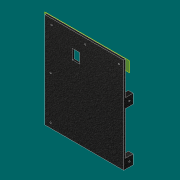
# Autodesk Inventor part: Lateral Derecho
Saved by Autodesk Inventor 2019 (Build 230136000, 136)
## iProperties
Created: 2024-12-30
Part Number: Lateral Derecho
Material: Nylon 6/6
Document SubType Name: Modeling
Designer: Familia CS
Density: 1.13 g/cm^3
Appearance: Black Cast
Author: Familia CS
Autodesk Inventor part; units mm, degrees
ref_plane "YZ Plane" through (0, 0, 0) normal (1, 0, 0) x (0, 1, 0)
ref_plane "XZ Plane" through (0, 0, 0) normal (0, 1, 0) x (-1, 0, 0)
ref_plane "XY Plane" through (0, 0, 0) normal (0, 0, 1) x (1, 0, 0)
ref_plane "Work Plane1" through (0, 0, 0) normal (0, 0, 1) x (1, 0, 0)
sketch "Sketch1" plane through (0, 0, 0) normal (0, 0, 1) x (1, 0, 0)
  line L0 (-2, -98) -> (8, -98) projected
  line L1 (-2, -98) -> (-2, 2) projected
  circle A0 centre (4, -93) radius 0.75 projected
  circle A1 centre (4, -48) radius 0.75 projected
  circle A2 centre (5, -4) radius 0.75 projected
  line L2 (0, 2) -> (80.5, 2) projected
  circle A3 centre (40.25, -4) radius 0.75 projected
  circle A4 centre (75.5, -4) radius 0.75 projected
  line L3 (34.223, -24.7194) -> (34.223, -14.2194)
  line L4 (26.723, -24.7194) -> (34.223, -24.7194)
  line L5 (26.723, -14.2194) -> (26.723, -24.7194)
  line L6 (34.223, -14.2194) -> (26.723, -14.2194)
  line L7 (80.5, 2) -> (-2, 2)
  line L8 (-2, 2) -> (-2, -98)
  line L9 (-2, -98) -> (80.5, -98)
  line L10 (80.5, -98) -> (80.5, 2)
  point P0 (0, 0)
  point P1 (20.6901, -14.1894)
  constraints: 16 end point, 3 horizontal, 2 parallel, 2 vertical, 1 perpendicular, 5 other
extrude "Extrusion1" add sketch "Sketch1" along normal blind 2
sketch "Sketch2" plane through (0, 0, 0) normal (0, 0, -1) x (-1, 0, 0)
  point P0 (0, 0)
sketch "Sketch3" plane through (0, 0, 0) normal (0, 0, -1) x (-1, 0, 0)
  point P0 (0, 0)
sketch "Sketch4" plane through (80.5, -98, 0) normal (1, 0, 0) x (0, 0, -1)
  line L0 (0, 45) -> (0, 55) projected
  line L1 (0, 45) -> (5, 45) projected
  line L2 (5, 55) -> (5, 45) projected
  line L3 (0, 55) -> (5, 55) projected
  line L4 (0, 45) -> (8, 45)
  line L5 (8, 45) -> (8, 55)
  line L6 (8, 55) -> (0, 55)
  circle A0 centre (4, 50) radius 0.75
  point P0 (0, 98)
  dimension "d3" = 8
  dimension "d4" = 10
  dimension "d6" = 1.5
  constraints: 6 end point, 1 centre point, 1 horizontal, 1 perpendicular
  measures "d3" distance of L0.start L4.end
  measures "d4" distance of L4.end L5.end
  measures "d6" diameter of A0
extrude "Extrusion2" add sketch "Sketch4" against normal blind 5
sketch "Sketch5" plane through (80.5, -98, 2) normal (1, 0, 0) x (0, 0, -1)
  line L0 (2, 45) -> (2, 0) projected
  line L1 (2, 0) -> (10, 0)
  line L2 (10, 0) -> (10, 10)
  line L3 (10, 10) -> (2, 10)
  line L4 (2, 10) -> (2, 0)
  circle A0 centre (6, 5) radius 0.75
  point P0 (2, 98)
  dimension "d9" = 8
  dimension "d10" = 10
  dimension "d12" = 1.5
  constraints: 8 end point, 2 parallel, 1 centre point, 1 horizontal, 1 perpendicular
  measures "d9" distance of L3.end L2.end
  measures "d10" distance of L2.end L1.end
  measures "d12" diameter of A0
extrude "Extrusion3" add sketch "Sketch5" against normal blind 5
sketch "Sketch6" plane through (-2, -98, 2) normal (0, -1, 0) x (1, 0, 0)
  line L0 (77.5, -10) -> (77.5, -2) projected
  line L1 (77.5, -10) -> (67.5, -10)
  line L2 (67.5, -10) -> (67.5, -2)
  line L3 (67.5, -2) -> (77.5, -2)
  line L4 (77.5, -2) -> (77.5, -10)
  circle A0 centre (72.5, -6) radius 0.75
  point P0 (2, -2)
  dimension "d15" = 10
  dimension "d16" = 8
  dimension "d18" = 1.5
  constraints: 8 end point, 2 parallel, 1 centre point, 1 horizontal, 1 perpendicular
  measures "d15" distance of L2.end L3.end
  measures "d16" distance of L1.end L2.end
  measures "d18" diameter of A0
extrude "Extrusion4" add sketch "Sketch6" against normal blind 5
sketch "Sketch7" plane through (-2, -98, 2) normal (0, -1, 0) x (1, 0, 0)
  line L0 (10, -2) -> (10, -17) projected
  line L1 (67.5, -10) -> (67.5, -2) projected
  circle A0 centre (32.473, -6) radius 0.75
  line L2 (32.473, -10) -> (27.473, -10)
  line L3 (27.473, -10) -> (27.473, -2)
  line L4 (27.473, -2) -> (37.473, -2)
  line L5 (37.473, -2) -> (37.473, -10)
  line L6 (37.473, -10) -> (32.473, -10)
  point P0 (2, -2)
  dimension "d22" = 1.5
  dimension "d25" = 4
  dimension "d26" = 5
  dimension "d27" = 8
  dimension "d28" = 10
  dimension "d29" = 8
  constraints: 10 end point, 2 perpendicular, 1 centre point, 1 point on line
  measures "d22" diameter of A0
  measures "d25" distance of A0.centre L2.start
  measures "d26" distance of L2.start L2.end
  measures "d27" distance of L2.end L3.end
  measures "d28" distance of L3.end L4.end
  measures "d29" distance of L4.end L5.end
extrude "Extrusion5" add sketch "Sketch7" against normal blind 5
sketch "Sketch8" plane through (-2, -98, 2) normal (0, -1, 0) x (1, 0, 0)
  line L0 (37.473, -10) -> (27.473, -10) projected
  line L1 (27.473, -10) -> (37.473, -10)
  line L2 (37.473, -10) -> (37.473, -2)
  line L3 (37.473, -2) -> (27.473, -2)
  line L4 (27.473, -2) -> (27.473, -10)
  point P0 (2, -2)
  constraints: 8 end point, 2 parallel, 1 horizontal, 1 perpendicular
extrude "Extrusion6" cut sketch "Sketch8" against normal blind 5
sketch "Sketch9" plane through (-2, -98, 2) normal (0, -1, 0) x (1, 0, 0)
  line L0 (47.25, -2) -> (47.25, -7) projected
  line L1 (47.25, -7) -> (37.25, -7) projected
  line L2 (37.25, -7) -> (37.25, -2) projected
  line L3 (37.25, -2) -> (47.25, -2)
  line L4 (67.5, -2) -> (0, -2) projected
  line L5 (37.25, -2) -> (37.25, -10)
  line L6 (37.25, -10) -> (47.25, -10)
  line L7 (47.25, -10) -> (47.25, -2)
  line L8 (47.25, -2) -> (37.25, -2)
  circle A0 centre (42.25, -6) radius 0.75
  point P0 (2, -2)
  dimension "d35" = 8
  dimension "d36" = 10
  dimension "d38" = 1.5
  constraints: 10 end point, 2 collinear, 1 centre point, 1 perpendicular, 1 vertical
  measures "d35" distance of L2.end L5.end
  measures "d36" distance of L5.end L6.end
  measures "d38" diameter of A0
extrude "Extrusion7" add sketch "Sketch9" against normal blind 5
sketch "Sketch10" plane through (80.5, -53, -8) normal (0, 0, -1) x (-1, 0, 0)
  line L0 (5, 10) -> (5, 0) projected
  line L1 (0, -45) -> (0, 55) projected
  line L2 (5, 0) -> (0, 0)
  line L3 (0, 0) -> (0, 10)
  line L4 (0, 10) -> (5, 10)
  line L5 (5, 10) -> (5, 0)
  point P0 (80.5, 53)
  dimension "d41" = 10
  constraints: 8 end point, 2 parallel, 1 horizontal, 1 perpendicular, 1 point on line
  measures "d41" distance of L2.end L3.end
extrude "Extrusion8" cut sketch "Sketch10" against normal blind 8
sketch "Sketch11" plane through (0, 0, 0) normal (0, 0, -1) x (-1, 0, 0)
  circle A0 centre (-4, -48) radius 0.75 projected
  line L0 (-80.5, 2) -> (-80.5, -88) projected
  line L1 (-80.5, -48) -> (-80.5, -43)
  line L2 (-80.5, -43) -> (-80.5, -33)
  line L3 (-80.5, -33) -> (-75.5, -33)
  line L4 (-75.5, -33) -> (-75.5, -43)
  line L5 (-75.5, -43) -> (-80.5, -43)
  point P0 (0, 0)
  dimension "d44" = 5
  dimension "d45" = 10
  dimension "d46" = 5
  dimension "d47" = 10
  constraints: 10 end point, 2 perpendicular, 2 point on line, 1 midpoint
  measures "d44" distance of L1.start L1.end
  measures "d45" distance of L1.end L2.end
  measures "d46" distance of L2.end L3.end
  measures "d47" distance of L3.end L4.end
extrude "Extrusion9" add sketch "Sketch11" along normal blind 8 contours L3 L4 L5 L0
sketch "Sketch12" plane through (80.5, -98, 2) normal (1, 0, 0) x (0, 0, -1)
  line L0 (10, 65) -> (10, 55) projected
  circle A0 centre (6, 60) radius 0.75
  point P0 (2, 98)
  dimension "d51" = 1.5
  constraints: 1 centre point
  measures "d51" diameter of A0
extrude "Extrusion10" cut sketch "Sketch12" against normal blind 5
body "Solid1"
